skadis_nut_left (Autodesk Fusion 360 design; units mm, degrees)
part number: 2026-09-06-14-40-21-794
Autodesk Fusion 360 part; units mm, degrees
sketch "Plate" plane through (0, 0, 0) normal (0, 1, 0) x (1, 0, 0)
  line L0 (0, 0) -> (11, 0)
  line L1 (11, 0) -> (11, -48)
  line L2 (11, -48) -> (0, -48)
  line L3 (0, -48) -> (0, 0)
  dimension "d271" = 11
  dimension "d272" = 48
  constraint coincident L0.start L3.end
  constraint horizontal L0
  constraint horizontal L2
  constraint vertical L1
  constraint vertical L3
  measures "d271" horizontal distance of L0.start L1.end
  measures "d272" vertical distance of L0.start L1.end
extrude "Plate (1)" add sketch "Plate" along normal mid plane 33 from surface at 4.5
sketch "Hook profile" plane through (0, 0, 0) normal (0, 1, 0) x (1, 0, 0)
  line L0 (0, -46) -> (-8.3, -46)
  line L1 (-8.3, -46) -> (-8.3, -29)
  line L2 (-8.3, -29) -> (-5.3, -29)
  line L3 (-5.3, -29) -> (-3.8, -30.5)
  line L4 (-3.8, -30.5) -> (-3.8, -41)
  line L5 (-3.8, -41) -> (0, -41)
  line L6 (0, -41) -> (0, -46)
  dimension "d276" = 46
  dimension "d277" = 8.3
  dimension "d278" = 3.8
  dimension "d279" = 5
  dimension "d280" = 10.5
  dimension "d281" = 1.5
  dimension "d282" = 1.5
  constraint horizontal L0
  constraint horizontal L2
  constraint horizontal L5
  constraint vertical L1
  constraint vertical L4
  constraint vertical L6
  constraint coincident origin L6
  measures "d276" vertical distance of origin L0.start
  measures "d277" horizontal distance of L0.start L0.end
  measures "d278" horizontal distance of L4.end L5.end
  measures "d279" vertical distance of L0.start L5.end
  measures "d280" vertical distance of L3.end L4.end
  measures "d281" horizontal distance of L2.end L3.end
  measures "d282" vertical distance of L2.end L3.end
extrude "Hook profile (1)" add sketch "Hook profile" along normal mid plane 2.4
pattern_linear "Hook rows" count 2 spacing 25.4 along (0, 0, -1) count 3 spacing 0 along (0, 0, 1) of "Hook profile (1)"
sketch "Screw hole" plane through (0, 0, 0) normal (0, 1, 0) x (1, 0, 0)
  line L0 (-1, -21.6) -> (12, -21.6)
  line L1 (12, -21.6) -> (12, -26.4)
  line L2 (12, -26.4) -> (-1, -26.4)
  line L3 (-1, -26.4) -> (-1, -21.6)
  dimension "d289" = 12
  dimension "d290" = 21.6
  dimension "d291" = 13
  dimension "d292" = 4.8
  constraint horizontal L0
  constraint horizontal L2
  constraint vertical L1
  constraint vertical L3
  measures "d289" horizontal distance of origin L0.end
  measures "d290" vertical distance of origin L0.end
  measures "d291" horizontal distance of L0.start L0.end
  measures "d292" vertical distance of L0.end L1.end
extrude "Screw hole (1)" cut sketch "Screw hole" along normal mid plane 16.8 from surface at 7.52
sketch "Nut cavity" plane through (0, 0, 0) normal (0, 1, 0) x (1, 0, 0)
  line L0 (3.6, -20.3) -> (7, -20.3)
  line L1 (7, -20.3) -> (7, -27.7)
  line L2 (7, -27.7) -> (3.6, -27.7)
  line L3 (3.6, -27.7) -> (3.6, -20.3)
  dimension "d296" = 7
  dimension "d297" = 20.3
  dimension "d298" = 3.4
  dimension "d299" = 7.4
  constraint horizontal L0
  constraint horizontal L2
  constraint vertical L1
  constraint vertical L3
  measures "d296" horizontal distance of origin L0.end
  measures "d297" vertical distance of origin L0.end
  measures "d298" horizontal distance of L0.start L0.end
  measures "d299" vertical distance of L0.end L1.end
extrude "Nut cavity (1)" cut sketch "Nut cavity" along normal mid plane 30.22 from surface at 2.11
equation "bracketWidth = 24.0 mm" comment "bracket width across the upright"
equation "plateHeight = 48.0 mm" comment "plate height"
equation "plateInboardExtension = 9.0 mm" comment "extra plate toward the desk centre, where the channel reaches"
equation "boardThickness = 6.0 mm" comment "measured SKADIS panel thickness"
equation "screwLength = 15.0 mm" comment "measured decorative M4 screw"
equation "screwDiameter = 4.0 mm" comment "M4 shank"
equation "screwClearance = 0.8 mm" comment "slack around the shank"
equation "screwTipClearance = 2.0 mm" comment "tip stops this short of the plate's back face"
equation "screwSlotWidth = screwDiameter + screwClearance" comment "screw relief slot height"
equation "nutAcrossFlats = 7.0 mm" comment "M4 square nut across flats"
equation "nutThickness = 3.0 mm" comment "M4 square nut thickness"
equation "nutChannelClearance = 0.4 mm" comment "slack around the nut in its channel"
equation "nutChannelHeight = nutAcrossFlats + nutChannelClearance" comment "channel height; under the nut's diagonal so it cannot turn"
equation "plateThickness = screwLength - boardThickness + screwTipClearance" comment "derived: deep enough to swallow the screw"
equation "mountTravel = 12.0 mm" comment "left-right adjustment"
equation "nutChannelLength = mountTravel + nutAcrossFlats + nutChannelClearance" comment "channel length along the plate"
equation "screwSlotLength = mountTravel + screwSlotWidth" comment "relief slot length along the plate"
equation "topMountZ = 24.0 mm" comment "top channel centre"
equation "mountOffsetY = 7.52 mm" comment "channel centre on the board's grid"
equation "slotOvershoot = 1.0 mm" comment "cuts reach past the faces they cut"
equation "slotWidth = 3.2 mm" comment "measured upright slot width"
equation "slotPitchVertical = 25.4 mm" comment "1 inch, measured"
equation "faceMetalThickness = 2.0 mm" comment "upright face metal"
equation "hookTabWidth = slotWidth - 0.8 mm" comment "blade width through the slot"
equation "hookThroat = faceMetalThickness + 1.8 mm" comment "gap behind the plate"
equation "hookNeckHeight = 5.0 mm" comment "bears on the slot bottom edge"
equation "hookLipThickness = 4.5 mm" comment "lip behind the upright face"
equation "hookLipDrop = 12.0 mm" comment "engagement below the neck"
equation "hookLipChamfer = 1.5 mm" comment "lead-in past slot burrs"
equation "topHookNeckTop = plateHeight - 2 mm" comment "top hook row"
equation "hookRows = 2" comment "hook rows (pattern count)"
equation "nutCavityClearance = 0.4 mm" comment "slack across the nut's thickness"
equation "nutWallThickness = 4.0 mm" comment "wall in front of the nut; the screw pulls the nut against it"
equation "nutCavityDepth = nutThickness + nutCavityClearance" comment "cavity depth"
equation "d271 = plateThickness"
equation "d272 = plateHeight"
equation "d273 = plateInboardExtension / 2"
equation "d274 = bracketWidth + plateInboardExtension"
equation "d276 = topHookNeckTop"
equation "d277 = hookThroat + hookLipThickness"
equation "d278 = hookThroat"
equation "d279 = hookNeckHeight"
equation "d280 = hookLipDrop - hookLipChamfer"
equation "d281 = hookLipChamfer"
equation "d282 = hookLipChamfer"
equation "d283 = hookTabWidth"
equation "d285 = hookRows"
equation "d287 = -slotPitchVertical"
equation "d289 = plateThickness + slotOvershoot"
equation "d290 = topMountZ - screwSlotWidth / 2"
equation "d291 = plateThickness + 2 * slotOvershoot"
equation "d292 = screwSlotWidth"
equation "d293 = mountOffsetY"
equation "d294 = screwSlotLength"
equation "d296 = plateThickness - nutWallThickness"
equation "d297 = topMountZ - nutChannelHeight / 2"
equation "d298 = nutCavityDepth"
equation "d299 = nutChannelHeight"
equation "d300 = ( mountOffsetY + nutChannelLength / 2 - bracketWidth / 2 - slotOvershoot ) / 2"
equation "d301 = mountOffsetY + nutChannelLength / 2 + bracketWidth / 2 + slotOvershoot"
named bodies: "skadis_nut_left"
